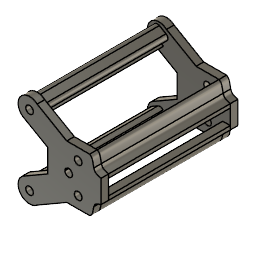
ION-Truster(150,2.5) (Autodesk Fusion 360 design; units mm, degrees)
Autodesk Fusion 360 part; units mm, degrees
sketch "Sketch1" plane through (0, 0, 0) normal (0, 1, 0) x (1, 0, 0) in component "ION-Truster(140,3.5) v7"
  line L0 (25, -50) -> (55, -50)
  line L1 (70, -14.9997) -> (70, -30)
  arc A0 (-13.9711, 42.5006) -> (-33.7134, 19.4647) centre (-23.8951, 31.0279) ccw
  spline S0 degree 2 poles (70, -30) (62.2402, -32.4595) (60.5, -37) knots 0 0 0 1.246987 1.246987 1.246987 weights 1 3 1
  circle A1 centre (-23.8951, -61.0274) radius 5
  line L2 (60, -30) -> (55, -30)
  line L3 (0, -29.9997) -> (-33.7134, -49.4642)
  line L4 (70, -14.9997) -> (70, 0.0006)
  circle A2 centre (40, 5.0006) radius 5
  line L5 (55, -50) -> (55, -30)
  line L6 (0, 0.0003) -> (-33.7134, 19.4647)
  line L7 (75, -14.9997) -> (70, -14.9997)
  arc A3 (-33.7134, -49.4642) -> (-13.9711, -72.5) centre (-23.8951, -61.0274) ccw
  line L8 (60, 0.0006) -> (55, 0.0006)
  spline S1 degree 2 poles (55, -50) (58.4982, -47.548) (60.5, -37) knots 0 0 0 1.457598 1.457598 1.457598 weights 1 3 1
  line L9 (55, 20.0006) -> (55, 0.0006)
  spline S2 degree 2 poles (55, 20.0006) (58.4982, 17.5486) (60.5, 7.0006) knots 0 0 0 1.457598 1.457598 1.457598 weights 1 3 1
  line L10 (0, -29.9997) -> (0, -14.9997)
  spline S3 degree 2 poles (70, 0.0006) (62.2402, 2.4601) (60.5, 7.0006) knots 0 0 0 1.246987 1.246987 1.246987 weights 1 3 1
  line L11 (75, -14.9997) -> (-15, -14.9997) construction
  line L12 (60, 0.0006) -> (60, -14.9997)
  line L13 (70, -14.9997) -> (70, -30)
  line L14 (25, 20.0006) -> (55, 20.0006)
  line L15 (25, 20.0006) -> (-13.9711, 42.5006)
  line L16 (25, -50) -> (-13.9711, -72.5)
  arc A4 (22.5, -14.9997) -> (32.5, -14.9997) centre (27.5, -15) ccw
  arc A5 (32.5, -14.9997) -> (22.5, -14.9997) centre (27.5, -14.9994) ccw
  line L17 (0, 0.0003) -> (0, -14.9997)
  circle A6 centre (40, -35) radius 5
  line L18 (60, -30) -> (60, -14.9997)
  circle A7 centre (-23.8951, 31.0279) radius 5
  point P0 (60.5, -37)
  dimension "d81" = 70
  dimension "d82" = 30
  dimension "d83" = 7
  dimension "d84" = 150
  dimension "d85" = 45
  dimension "d86" = 10
  dimension "d87" = 10
  dimension "d88" = 10
  dimension "d89" = 15
  dimension "d90" = 42.5
  dimension "d91" = 30
  dimension "d92" = 15
  dimension "d93" = 35
  constraint vertical L1
  constraint vertical L10
  constraint horizontal L0
  constraint coincident P0 S0.end
  constraint perpendicular L1 L7
  constraint parallel L3 L16
  constraint concentric A1 A3
  constraint vertical L18
  constraint vertical L13
  constraint perpendicular L0 L5
  constraint perpendicular L10 L11
  constraint coincident L10.end L11
  constraint coincident A4.end L11
  constraint coincident A4.start L11
  constraint coincident L12.end L11
  constraint symmetric L1.start L4.start L7
  constraint symmetric A0.end L3.end L7
  constraint symmetric L8.end L2.end L7
  constraint symmetric S2.end P0 L7
  constraint symmetric L6.start L3.start L7
  constraint symmetric L4.end L1.end L7
  constraint symmetric L0.end L9.start L7
  constraint symmetric L0.start L14.start L7
  constraint symmetric L8.start L2.start L7
  constraint symmetric A3.end A0.start L7
  constraint symmetric L7 S1 S2
  constraint symmetric A2 L7 A6
  constraint symmetric A0 L7 A3
  constraint symmetric S0 L7 S3
  constraint symmetric L10.end L17.end L7
  constraint symmetric A4.end A5.start L7
  constraint symmetric A4.start A5.end L7
  constraint symmetric L7 A4 A5
  constraint symmetric L12.end L18.end L7
  constraint symmetric A1 L7 A7
  measures "d81" distance of L3.start L1.end
  measures "d82" distance of L0.start L0.end
  measures "d83" vertical distance of L1.end P0
  measures "d84" angle of L0 L16
  measures "d85" distance of L0.start A3.end
  measures "d86" diameter of A1
  measures "d87" diameter of A6
  measures "d88" diameter of A4
  measures "d89" distance of A6.centre L0
  measures "d90" distance of A4.centre L1
  measures "d91" distance of A6.centre L1
  measures "d92" distance of L10.end L3.start
  measures "d93" distance of A4.centre L0
extrude "Extrude1" add sketch "Sketch1" against normal blind 10 makes body 1 in component "ION-Truster(140,3.5) v7"
extrude "Extrude2" add sketch "Sketch1" along normal blind 160 separate body contours L1 S0 L2 L4 L5 L8 S1 L9 S2 S3 L12 L13 L18 makes body 2 in component "ION-Truster(140,3.5) v7"
copy_body "CopyPasteBodies1" bodies 1 makes body 3 in component "ION-Truster(140,3.5) v7"
move_body "Move1" bodies 3 to x (1, 0, 0) y (0, 1, 0) z (0, 0, 1) at (0, 170, 0) in component "ION-Truster(140,3.5) v7"
sketch "Sketch2" plane through (70, 0, 0) normal (1, 0, 0) x (0, 1, 0) in component "ION-Truster(140,3.5) v7"
  line L0 (0, 30) -> (0, 0)
  line L1 (0, 0) -> (160, 0)
  line L2 (160, 0) -> (160, 30)
  line L3 (160, 30) -> (0, 30)
  line L4 (0, 25) -> (160, 25)
  line L5 (160, 25) -> (160, 5)
  line L6 (160, 5) -> (0, 5)
  line L7 (0, 5) -> (0, 25)
  dimension "d36" = 5
  dimension "d37" = 5
  dimension "d99" = 160
  constraint horizontal L4
  constraint vertical L5
  constraint horizontal L6
  constraint vertical L7
  constraint coincident L2 L5.end
  constraint coincident L0 L4.start
  measures "d36" distance of L3 L4
  measures "d37" distance of L1 L6
  measures "d99" distance of L5 L7
extrude "Extrude3" cut sketch "Sketch2" against normal up to surface (10 mm away) contours L0 L2 L4 L5 L6 L7 bodies 2 makes body 4 at (55, 53.3333, 43.3333) in component "ION-Truster(140,3.5) v7"
sketch "Sketch3" plane through (0, 160, 0) normal (0, -1, 0) x (1, 0, 0) in component "ION-Truster(140,3.5) v7"
  line L0 (-27.6336, 74.748) -> (-10.3251, 64.7248)
  line L1 (-10.3251, 64.7248) -> (-20.0962, 47.4139)
  line L2 (-20.0962, 47.4139) -> (-37.525, 57.2238)
  line L3 (-37.525, 57.2238) -> (-27.6336, 74.748)
  circle A0 centre (-23.8951, -31.0279) radius 5
  arc A1 (22.5, 14.9997) -> (32.5, 14.9997) centre (27.5, 14.9994) ccw
  arc A2 (32.5, 14.9997) -> (22.5, 14.9997) centre (27.5, 15) ccw
  circle A3 centre (40, -5.0006) radius 5
  circle A4 centre (40, 35) radius 5
  circle A5 centre (-23.8951, 61.0274) radius 5
  line L4 (-13.9711, -42.5006) -> (25, -20.0006)
  line L5 (25, -20.0006) -> (55, -20.0006)
  spline S0 degree 2 poles (55, -20.0006) (58.4982, -17.5486) (60.5, -7.0006) knots 0 0 0 1.457598 1.457598 1.457598 weights 1 3 1
  spline S1 degree 2 poles (60.5, -7.0006) (62.2402, -2.4601) (70, -0.0006) knots -1.246987 -1.246987 -1.246987 0 0 0 weights 1 3 1
  line L6 (70, -0.0006) -> (70, 30)
  spline S2 degree 2 poles (70, 30) (62.2402, 32.4595) (60.5, 37) knots 0 0 0 1.246987 1.246987 1.246987 weights 1 3 1
  spline S3 degree 2 poles (60.5, 37) (58.4982, 47.548) (55, 50) knots -1.457598 -1.457598 -1.457598 0 0 0 weights 1 3 1
  line L7 (55, 50) -> (25, 50)
  line L8 (25, 50) -> (-13.9711, 72.5)
  arc A6 (-13.9711, 72.5) -> (-33.7134, 49.4642) centre (-23.8951, 61.0274) ccw
  line L9 (-33.7134, 49.4642) -> (0, 29.9997)
  line L10 (0, 29.9997) -> (0, -0.0003)
  line L11 (0, -0.0003) -> (-33.7134, -19.4647)
  arc A7 (-33.7134, -19.4647) -> (-13.9711, -42.5006) centre (-23.8951, -31.0279) ccw
  point P0 (-23.8951, 61.0274)
  dimension "d40" = 10
  dimension "d41" = 10
  dimension "d42" = 20
  dimension "d43" = 10
  constraint coincident P0 A5.centre
  measures "d40" distance of L2 P0
  measures "d41" distance of L0 P0
  measures "d42" distance of L1 L3
  measures "d43" distance of L3 P0
extrude "Extrude4" add sketch "Sketch3" along normal blind 160 separate body contours L0 L1 L2 L3 | A5 makes body 5 in component "ION-Truster(140,3.5) v7"
sketch "Sketch5" plane through (-35.5367, 0, 20.0585) normal (0.870851, 0, -0.491547) x (0, 1, 0) in component "ION-Truster(140,3.5) v7"
  line L0 (160, 31.4122) -> (160, 51.2903)
  line L1 (160, 51.2903) -> (0, 51.2903)
  line L2 (0, 51.2903) -> (0, 31.4122)
  line L3 (0, 31.4122) -> (160, 31.4122)
  line L4 (0, 46.7903) -> (160, 46.7903)
  line L5 (160, 46.7903) -> (160, 35.9122)
  line L6 (160, 35.9122) -> (0, 35.9122)
  line L7 (0, 35.9122) -> (0, 46.7903)
  dimension "d56" = 4.5
  dimension "d57" = 4.5
  constraint horizontal L4
  constraint vertical L5
  constraint horizontal L6
  constraint vertical L7
  constraint coincident L0 L5.end
  constraint coincident L2 L4.start
  measures "d56" distance of L1 L4
  measures "d57" distance of L3 L6
extrude "Extrude7" cut sketch "Sketch5" against normal blind 10 contours L0 L2 L4 L5 L6 L7 bodies 5 in component "ION-Truster(140,3.5) v7"
copy_body "CopyPasteBodies2" bodies 5 makes body 6 in component "ION-Truster(140,3.5) v7"
move_body "Move2" bodies 6 to x (1, 0, 0) y (0, 1, 0) z (0, 0, 1) at (7, 0, -91) in component "ION-Truster(140,3.5) v7"
move_body "Move5" bodies 6 to x (0.5, 0, 0.866025) y (0, 1, 0) z (-0.866025, 0, 0.5) at (-41.908, 0, -1.6088) in component "ION-Truster(140,3.5) v7"
fillet "Fillet3" radius 5 8 edges at (-27.6336, 80, 74.748) (-37.525, 80, 57.2238) (-20.0962, 80, 47.4139) (-10.3251, 80, 64.7248) (-38.1502, 80, -27.604) (-20.8156, 80, -17.6261) (-10.7094, 80, -34.7435) (-27.9195, 80, -44.9324) on bodies 5 6 in component "ION-Truster(140,3.5) v7"
fillet "Fillet4" [suppressed] in component "ION-Truster(140,3.5) v7"
component "ION-Truster(140,3.5) v7" placed x (1, 0, 0) y (0, 1, 0) z (0, 0, 1) at (0, 0, 0)
equation "d41 = d40"
equation "Angle = ( ( 150 cm ) / cm ) * 1 deg" comment "angle of the arms"
equation "distance = 3 cm" comment "distance of the first 2 holes"
equation "d84 = Angle"
equation "d90 = distance + 1.25 cm"
equation "d91 = distance"
